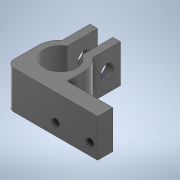
# Autodesk Inventor part: zstop
Saved by Autodesk Inventor 2020.2 (Build 242310000, 310)
## iProperties
Created: 2020-08-09
Part Number: zstop
Material: Generic
Document SubType Name: Modeling
Designer: JK
Density: 1 g/cm^3
Appearance: Smooth - Black
Author: JK
Autodesk Inventor part; units mm, degrees
ref_plane "YZ Plane" through (0, 0, 0) normal (1, 0, 0) x (0, 1, 0)
ref_plane "XZ Plane" through (0, 0, 0) normal (0, 1, 0) x (-1, 0, 0)
ref_plane "XY Plane" through (0, 0, 0) normal (0, 0, 1) x (1, 0, 0)
sketch "Sketch1" plane through (0, 0, 0) normal (0, 1, 0) x (-1, 0, 0)
  circle A0 centre (0, 0) radius 4.25
  circle A1 centre (0, 0) radius 6
  line L0 (6, 0) -> (-6, 0)
  line L1 (-6, 0) -> (-6, 8.25)
  line L2 (-6, 8.25) -> (6, 8.25)
  line L3 (6, 8.25) -> (6, 0)
  line L4 (6, 8.25) -> (-18, 8.25)
  line L5 (-18, 8.25) -> (-18, 4.25)
  line L6 (-18, 4.25) -> (6, 4.25)
  line L7 (6, 4.25) -> (6, 8.25)
  point P0 (-4.2353, 4.25)
  point P1 (4.2353, 4.25)
  point P2 (6, 8.25)
  point P3 (-6, 4.25)
  point P4 (6, 4.25)
  dimension "d1" = 12
  dimension "d0" = 8.5
  dimension "d2" = 4
  dimension "d3" = 6
  dimension "d4" = 18
  constraints: 16 end point, 4 parallel, 2 coincident, 2 horizontal, 2 perpendicular, 1 centre point, 1 point on line, 1 vertical, 3 other
  measures "d0" diameter of A0
  measures "d2" distance between parallel lines of L6 L4
  measures "d3" distance from line of L7 point (0, 0)
  measures "d4" distance from line of point (0, 0) L5
extrude "Extrusion1" add sketch "Sketch1" along normal blind 10 contours L0 A1 A0 | A0 L6 A1 L0 | A0 L0 A1 L6 | L6 A1 | A1 L6 L3 | L6 L1 L2 L3 A1 | A1 L1 L6 | L6 L5 L4 L1
sketch "Sketch2" plane through (0, 10, 0) normal (0, 1, 0) x (1, 0, 0)
  line L0 (-2, 1.8795) -> (2, 1.8795)
  line L1 (2, 1.8795) -> (2, 9.0075)
  line L2 (2, 9.0075) -> (-2, 9.0075)
  line L3 (-2, 9.0075) -> (-2, 1.8795)
  point P0 (0, 0)
  dimension "d7" = 2
  dimension "d8" = 2
  constraints: 8 end point, 2 parallel, 1 horizontal, 1 perpendicular
  measures "d7" distance from line of point (0, 0) L3
  measures "d8" distance from line of L1 point (0, 0)
extrude "Extrusion2" cut sketch "Sketch2" against normal blind 10
sketch "Sketch3" plane through (0, 10, 0) normal (0, 1, 0) x (1, 0, 0)
  line L0 (2, 3.75) -> (2, 5.6569) projected
  line L1 (2, 3.75) -> (4, 3.75)
  line L2 (4, 3.75) -> (4, 11.75)
  line L3 (4, 11.75) -> (2, 11.75)
  line L4 (2, 11.75) -> (2, 3.75)
  line L5 (-2, 3.75) -> (-2, 5.6569) projected
  line L6 (-2, 3.75) -> (-4, 3.75)
  line L7 (-4, 3.75) -> (-4, 11.75)
  line L8 (-4, 11.75) -> (-2, 11.75)
  line L9 (-2, 11.75) -> (-2, 3.75)
  point P0 (0, 0)
  dimension "d11" = 2
  dimension "d12" = 2
  dimension "d13" = 8
  dimension "d14" = 8
  constraints: 16 end point, 4 parallel, 2 horizontal, 2 perpendicular
  measures "d11" distance of L7.end L8.end
  measures "d12" distance of L2.end L3.end
  measures "d13" distance of L6.end L7.end
  measures "d14" distance of L1.end L2.end
extrude "Extrusion3" add sketch "Sketch3" against normal blind 10
sketch "Sketch4" plane through (4, 10, -4.4721) normal (1, 0, 0) x (0, 0, -1)
  circle A0 centre (3.7779, -5) radius 1.75
  line L0 (7.2779, 0) -> (7.2779, -10) projected
  point P0 (-4.4721, -10)
  dimension "d17" = 3.5
  dimension "d18" = 3.5
  constraints: 1 centre point
  measures "d17" diameter of A0
  measures "d18" distance from line of L0 A0.centre
extrude "Extrusion4" cut sketch "Sketch4" against normal through all
sketch "Sketch5" plane through (-6, 0, 8.25) normal (0, 0, 1) x (1, 0, 0)
  circle A0 centre (13, 3) radius 1
  circle A1 centre (22, 3) radius 1
  line L0 (0, 0) -> (0, 10) projected
  line L1 (0, 10) -> (24, 10) projected
  point P0 (6, 0)
  dimension "d21" = 2
  dimension "d22" = 9
  dimension "d24" = 7
  dimension "d27" = 16
  constraints: 2 centre point, 1 equal radius, 1 horizontal alignment
  measures "d21" diameter of A0
  measures "d22" distance of A1.centre A0.centre
  measures "d24" distance from line of L1 A0.centre
  measures "d27" horizontal distance of point (6, 0) A1.centre
extrude "Extrusion5" cut sketch "Sketch5" against normal through all
fillet "Fillet1" radius 2 1 edges at (-6, 5, 8.25)
body "Solid1"
